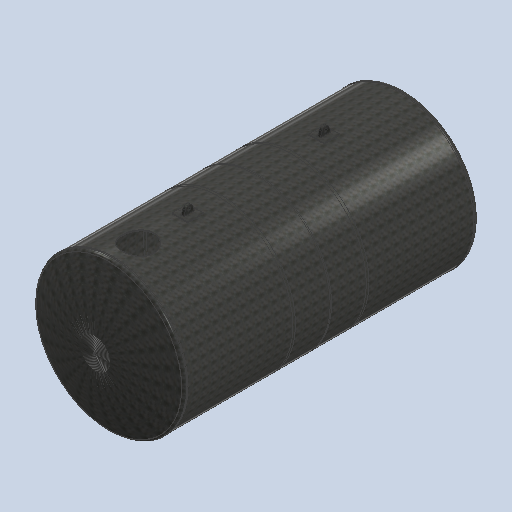
# Autodesk Inventor part: Tanque5000
Saved by Autodesk Inventor 2023 (Build 270158000, 158)
## iProperties
Created: 2022-11-02
Part Number: Tanque5000
Material: Steel ASTM A36
Document SubType Name: Modeling
Designer: Juanse
Density: 7.85 g/cm^3
Appearance: Plate
Author: Juanse
Autodesk Inventor part; units mm, degrees
ref_plane "YZ Plane" through (0, 0, 0) normal (1, 0, 0) x (0, 1, 0)
ref_plane "XY Plane" through (0, 0, 0) normal (0, 0, 1) x (1, 0, 0)
sketch "Sketch1" plane through (0, 0, 0) normal (0, 0, 1) x (1, 0, 0)
  circle A0 centre (0, 0) radius 1432.5
  circle A1 centre (0, 0) radius 1428
  circle A2 centre (0, 0) radius 1421
  circle A3 centre (0, 0) radius 1415
  dimension "d0" = 2865
  dimension "d1" = 4.5
  dimension "d2" = 6
  dimension "d5" = 2830
  constraints: 4 centre point, 4 coincident
  measures "d0" diameter of A0
  measures "d1" radial gap between concentric circles of A1 A0
  measures "d2" radial gap between concentric circles of A2 A3
  measures "d5" diameter of A3
extrude "Extrusion1" add sketch "Sketch1" along normal mid plane 5496
sketch "Sketch2" plane through (0, 0, 0) normal (1, 0, 0) x (0, 1, 0)
  line L0 (1421, -2748) -> (1421, 2748)
  line L1 (-1432.5, -2748) -> (1432.5, -2748)
  line L2 (1432.5, 2748) -> (-1432.5, 2748)
  line L3 (1428, 2748) -> (1428, -2748)
  line L4 (1432.5, -2748) -> (1432.5, 2748)
  line L5 (1415, 2748) -> (1415, -2748)
  line L6 (1421, 2748) -> (-1421, 2748)
  line L7 (0, 2748) -> (0, -2748)
  line L8 (1421, 2748) -> (1428, 2748)
  line L9 (1428, 2748) -> (1428, 2723)
  line L10 (1428, 2723) -> (1421, 2723)
  line L11 (1421, 2723) -> (1421, 2748)
  line L12 (-1421, -2748) -> (1421, -2748)
  line L13 (1421, -2748) -> (1428, -2748)
  line L14 (1428, -2748) -> (1428, -2723)
  line L15 (1428, -2723) -> (1421, -2723)
  line L16 (1421, -2723) -> (1421, -2748)
  line L17 (1421, 12.5) -> (1428, 12.5)
  line L18 (1428, 12.5) -> (1428, -12.5)
  line L19 (1428, -12.5) -> (1421, -12.5)
  line L20 (1421, -12.5) -> (1421, 12.5)
  line L21 (1421, 675) -> (1428, 675)
  line L22 (1428, 675) -> (1428, 725)
  line L23 (1428, 725) -> (1421, 725)
  line L24 (1421, 725) -> (1421, 675)
  line L25 (0, 0) -> (1421, 0) construction
  line L26 (1421, -675) -> (1428, -675)
  line L27 (1428, -675) -> (1428, -725)
  line L28 (1428, -725) -> (1421, -725)
  line L29 (1421, -725) -> (1421, -675)
  arc A0 (1432.5, 2748) -> (1391.524885, 2808.39706) centre (1367.5, 2748) ccw
  arc A1 (1391.524885, 2808.39706) -> (0, 3075) centre (0, -689.809637) ccw
  arc A2 (1389.861623, 2804.215726) -> (0, 3070.5) centre (0, -689.809637) ccw
  arc A3 (1428, 2748) -> (1389.861623, 2804.215726) centre (1367.5, 2748) ccw
  arc A4 (1387.274328, 2797.711427) -> (0, 3063.5) centre (0, -689.809637) ccw
  arc A5 (1421, 2748) -> (1387.274328, 2797.711427) centre (1367.5, 2748) ccw
  arc A6 (1385.056647, 2792.136313) -> (0, 3057.5) centre (0, -689.809637) ccw
  arc A7 (1415, 2748) -> (1385.056647, 2792.136313) centre (1367.5, 2748) ccw
  line L30 (25, 3063.416739) -> (25, 3070.416894)
  line L31 (0, 3075) -> (0, 3057.5)
  point P0 (1428, 0)
  point P1 (1428, 0)
  point P2 (1428, 700)
  point P3 (1428, -700)
  dimension "d12" = 25
  dimension "d13" = 25
  dimension "d14" = 25
  dimension "d15" = 50
  dimension "d16" = 700
  dimension "d24" = 65
  dimension "d25" = 327
  dimension "d28" = 25
  constraints: 48 end point, 19 point on circle, 8 centre point, 8 midpoint, 8 parallel, 8 tangent, 6 concentric, 6 point on line, 5 symmetric about line, 5 vertical alignment, 4 horizontal, 4 perpendicular, 2 vertical, 1 coincident
  measures "d12" distance of L8.end L9.end
  measures "d13" distance of L14.end L13.end
  measures "d14" distance of L17.end L18.end
  measures "d15" distance of L22.end L21.end
  measures "d16" distance of point (1428, 0) point (1428, 700)
  measures "d24" radius of A0
  measures "d25" distance from line of L2 L31.start
  measures "d28" distance between parallel lines of L31 L30
revolve "Revolution2" add sketch "Sketch2" angle 360 about axis through (0, 0, 2748) along (0, 0, -1) contours A7 A6 L31 A4 A5 L2 | L2 L3 L10 L0 | L2 A3 A2 L31 A1 A0 | L0 L17 L3 L19 | L23 L3 L21 L0 | A4 L31 A2 L30
mirror "Mirror1" about plane through (0, 0, 0) normal (0, 0, 1) of "Revolution2"
ref_plane "Work Plane1" through (0, 1432.5, 0) normal (0, 1, 0) x (-1, 0, 0)
sketch "Sketch3" plane through (0, 1432.5, 0) normal (0, 1, 0) x (-1, 0, 0)
  circle A0 centre (0, 2248) radius 305
  line L0 (1432.5, 2748) -> (-1432.5, 2748) projected
  point P0 (0, 0)
  dimension "d30" = 610
  dimension "d31" = 500
  constraints: 1 centre point
  measures "d30" diameter of A0
  measures "d31" distance from line of A0.centre L0
extrude "Extrusion2" cut sketch "Sketch3" against normal blind 100
sketch "Sketch4" plane through (0, 1432.5, 0) normal (0, 1, 0) x (-1, 0, 0)
  line L0 (-150, 1450) -> (150, 1450)
  line L1 (150, 1450) -> (150, 1150)
  line L2 (150, 1150) -> (-150, 1150)
  line L3 (-150, 1150) -> (-150, 1450)
  line L4 (-150, 1450) -> (150, 1150) construction
  line L5 (150, 1450) -> (-150, 1150) construction
  line L6 (0, 0) -> (0, 1300) construction
  point P0 (0, 650)
  dimension "d38" = 300
  dimension "d39" = 300
  dimension "d40" = 1300
  constraints: 14 end point, 4 midpoint, 2 coincident, 2 parallel, 1 horizontal, 1 perpendicular, 1 vertical
  measures "d38" distance of L1.end L2.end
  measures "d39" distance of L0.end L1.end
  measures "d40" distance of L6.start L6.end
extrude "Extrusion3" add sketch "Sketch4" along normal blind 6 and the other way blind 9
sketch "Sketch5" plane through (0, 0, 0) normal (1, 0, 0) x (0, 1, 0)
  line L0 (1424.624951, 1450) -> (1424.624951, 1150)
  line L1 (1424.624951, 1450) -> (1438.5, 1450)
  line L2 (1438.5, 1150) -> (1438.5, 1450)
  line L3 (1424.624951, 1150) -> (1438.5, 1150)
  line L4 (1438.5, 1150) -> (1438.5, 1450)
  line L5 (1438.5, 1400) -> (1534.5, 1372)
  arc A0 (1534.5, 1228) -> (1534.5, 1372) centre (1513.5, 1300) ccw
  line L6 (1534.5, 1228) -> (1438.5, 1200)
  circle A1 centre (1513.5, 1300) radius 30
  point P0 (0, 0)
  point P1 (1438.5, 1300)
  dimension "d45" = 100
  dimension "d46" = 100
  dimension "d47" = 75
  dimension "d48" = 200
  dimension "d49" = 60
  constraints: 4 end point, 2 centre point, 2 point on circle, 2 point on line, 2 tangent, 1 coincident, 1 horizontal alignment, 1 midpoint
  measures "d45" distance of L5.start L5.end
  measures "d46" distance of L6.start L6.end
  measures "d47" radius of A0
  measures "d48" distance of L6.end L5.start
  measures "d49" diameter of A1
extrude "Extrusion4" add sketch "Sketch5" along normal mid plane 50 contours L5 A0 L6 L2
mirror "Mirror2" about plane through (0, 0, 0) normal (0, 0, 1) of "Extrusion4", "Extrusion3"
equation "\"d12\" = d14"
equation "\"d13\" = d14"
equation "\"d15\" = 2 * d14"
equation "\"d28\" = d14"
body "Solid1"
